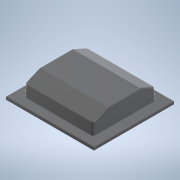
# Autodesk Inventor part: Case externa
Saved by Autodesk Inventor 2021 (Build 250183000, 183)
## iProperties
Created: 2023-04-12
Part Number: Case externa
Material: PPS Plastic
Document SubType Name: Modeling
Designer: Technolog35
Density: 1.637 g/cm^3
Appearance: Smooth - Black
Author: Technolog35
Autodesk Inventor part; units mm, degrees
ref_plane "YZ Plane" through (0, 0, 0) normal (1, 0, 0) x (0, 1, 0)
ref_plane "XZ Plane" through (0, 0, 0) normal (0, 1, 0) x (-1, 0, 0)
ref_plane "XY Plane" through (0, 0, 0) normal (0, 0, 1) x (1, 0, 0)
sketch "Base" plane through (0, 0, 0) normal (0, 1, 0) x (-1, 0, 0)
  line L0 (88.5, 80.5) -> (-88.5, 80.5)
  line L1 (-88.5, 80.5) -> (-88.5, -80.5)
  line L2 (-88.5, -80.5) -> (88.5, -80.5)
  line L3 (88.5, -80.5) -> (88.5, 80.5)
  line L4 (68, -61) -> (-68, -61)
  line L5 (-68, -61) -> (-68, 61)
  line L6 (-68, 61) -> (68, 61)
  line L7 (68, 61) -> (68, -61)
  line L8 (68, -61) -> (-68, 61) construction
  line L9 (-68, -61) -> (68, 61) construction
  point P0 (0, 0)
  point P1 (-88.5, 0)
  point P2 (0, -80.5)
  dimension "d0" = 177
  dimension "d1" = 161
  dimension "d25" = 136
  dimension "d26" = 122
  constraints: 20 end point, 4 midpoint, 3 parallel, 1 horizontal, 1 horizontal alignment, 1 perpendicular, 1 vertical alignment
  measures "d0" distance of L1.end L2.end
  measures "d1" distance of L0.end L1.end
  measures "d25" distance of L5.end L6.end
  measures "d26" distance of L4.end L5.end
extrude "Extrusion1" add sketch "Base" along normal blind 6 contours L3 L2 L1 L0 | L4 L5 L6 L7
sketch "Superior" plane through (0, 6, 0) normal (0, 1, 0) x (1, 0, 0)
  line L0 (-70, -63) -> (70, -63)
  line L1 (70, -63) -> (70, 63)
  line L2 (70, 63) -> (-70, 63)
  line L3 (-70, 63) -> (-70, -63)
  line L4 (-70, -63) -> (70, 63) construction
  line L5 (70, -63) -> (-70, 63) construction
  line L6 (68, -61) -> (-68, -61)
  line L7 (-68, -61) -> (-68, 61)
  line L8 (-68, 61) -> (68, 61)
  line L9 (68, 61) -> (68, -61)
  line L10 (68, -61) -> (-68, 61) construction
  line L11 (-68, -61) -> (68, 61) construction
  point P0 (0, 0)
  dimension "d7" = 140
  dimension "d8" = 126
  dimension "d23" = 136
  dimension "d24" = 122
  constraints: 24 end point, 4 midpoint, 4 parallel, 2 horizontal, 2 perpendicular
  measures "d7" distance of L2.end L1.end
  measures "d8" distance of L1.end L0.end
  measures "d23" distance of L7.end L8.end
  measures "d24" distance of L6.end L7.end
sketch "Superior outline for Extrusion2" plane through (0, 6, 0) normal (0, 1, 0) x (1, 0, 0)
  line L0 (-70, -63) -> (70, -63)
  line L1 (-70, 63) -> (-70, -63)
  line L2 (70, 63) -> (-70, 63)
  line L3 (70, -63) -> (70, 63)
extrude "Extrusion2" add sketch "Superior outline for Extrusion2" along normal blind 36 draft -2
chamfer "Top left" distance 13 distance2 29 1 edges at (0, 42, 61.7429) measured on face at (22.9143, 18, 62.581)
chamfer "Top right" distance 13 distance2 29 1 edges at (0, 42, -61.7429) measured on face at (-22.9143, 18, -62.581)
fillet "Fillet base" radius 1 4 edges at (88.5, 6, 0) (0, 6, 80.5) (0, 6, -80.5) (-88.5, 6, 0)
fillet "Fillet top" radius 2 2 edges at (0, 29.0079, -62.1965) (0, 29.0079, 62.1965)
fillet "Fillet top" radius 2 6 edges at (68.9697, 35.504, 47.4697) (68.7429, 42, 0) (68.9697, 35.504, -47.4697) (-68.9697, 35.504, 47.4697) (-68.7429, 42, 0) (-68.9697, 35.504, -47.4697)
fillet "Fillet top" radius 2 2 edges at (0, 42, 32.7429) (0, 42, -32.7429)
fillet "Fillet top" radius 1 4 edges at (0, 6, 63) (70, 6, 0) (0, 6, -63) (-70, 6, 0)
fillet "Fillet top" radius 5 4 edges at (69.5983, 17.504, 62.5983) (-69.5983, 17.504, 62.5983) (69.5983, 17.504, -62.5983) (-69.5983, 17.504, -62.5983)
sketch "Sketch8" plane through (0, 0, 0) normal (0, -1, 0) x (1, 0, 0)
  line L0 (-68, -61) -> (68, -61)
  line L1 (68, -61) -> (68, 61)
  line L2 (68, 61) -> (-68, 61)
  line L3 (-68, 61) -> (-68, -61)
  line L4 (-68, -61) -> (68, 61) construction
  line L5 (68, -61) -> (-68, 61) construction
  point P0 (0, 0)
  dimension "d27" = 136
  dimension "d28" = 122
  constraints: 12 end point, 2 midpoint, 2 parallel, 1 horizontal, 1 perpendicular
  measures "d27" distance of L2.end L1.end
  measures "d28" distance of L1.end L0.end
extrude "Extrusion3" cut sketch "Sketch8" against normal blind 28 draft -2
sketch "Sketch11" plane through (0, 0, 0) normal (0, -1, 0) x (1, 0, 0)
  line L0 (-85, -77) -> (85, -77)
  line L1 (85, -77) -> (85, 77)
  line L2 (85, 77) -> (-85, 77)
  line L3 (-85, 77) -> (-85, -77)
  line L4 (-85, -77) -> (85, 77) construction
  line L5 (85, -77) -> (-85, 77) construction
  point P0 (0, 0)
  dimension "d37" = 170
  dimension "d38" = 154
  constraints: 12 end point, 2 midpoint, 2 parallel, 1 horizontal, 1 perpendicular
  measures "d37" distance of L2.end L1.end
  measures "d38" distance of L1.end L0.end
extrude "Extrusion4" cut sketch "Sketch11" against normal blind 3.5
sketch "Sketch12" plane through (0, 28, 0) normal (0, -1, 0) x (1, 0, 0)
  line L0 (67.022218, 60.022218) -> (-67.022218, 60.022218)
  line L1 (-67.022218, -60.022218) -> (67.022218, -60.022218)
  line L2 (67.022218, -60.022218) -> (67.022218, 60.022218)
  line L3 (67.022218, 60.022218) -> (-67.022218, 60.022218)
  line L4 (-67.022218, 60.022218) -> (-67.022218, -60.022218)
  line L5 (-67.022218, -60.022218) -> (67.022218, 60.022218) construction
  line L6 (67.022218, -60.022218) -> (-67.022218, 60.022218) construction
  point P0 (0, 0)
  constraints: 12 end point, 2 midpoint, 2 parallel, 1 horizontal, 1 perpendicular
extrude "Extrusion5" cut sketch "Sketch12" against normal blind 12 draft -67
body "Solid1"
